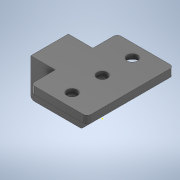
# Autodesk Inventor part: pulleysupport2
Saved by Autodesk Inventor 2020.2 (Build 242310000, 310)
## iProperties
Created: 2020-08-06
Part Number: pulleysupport2
Material: Generic
Document SubType Name: Modeling
Designer: JK
Density: 1 g/cm^3
Appearance: Smooth - Black
Author: JK
Autodesk Inventor part; units mm, degrees
ref_plane "YZ Plane" through (0, 0, 0) normal (1, 0, 0) x (0, 1, 0)
ref_plane "XZ Plane" through (0, 0, 0) normal (0, 1, 0) x (-1, 0, 0)
ref_plane "XY Plane" through (0, 0, 0) normal (0, 0, 1) x (1, 0, 0)
sketch "Sketch1" plane through (0, 0, 0) normal (0, 1, 0) x (-1, 0, 0)
  line L0 (-15, 23) -> (15, 23)
  line L1 (15, 23) -> (15, -23)
  line L2 (15, -23) -> (-15, -23)
  line L3 (-15, -23) -> (-15, 23)
  line L4 (-15, 23) -> (15, -23) construction
  line L5 (15, 23) -> (-15, -23) construction
  circle A0 centre (0, 16) radius 1.75
  circle A1 centre (0, -16) radius 1.75
  point P0 (0, 0)
  dimension "d0" = 3.5
  dimension "d1" = 30
  dimension "d2" = 46
  dimension "d3" = 16
  dimension "d4" = 16
  constraints: 12 end point, 2 centre point, 2 midpoint, 2 parallel, 1 equal radius, 1 horizontal, 1 perpendicular
  measures "d0" diameter of A0
  measures "d1" distance of L0.start L0.end
  measures "d2" distance of L0.end L1.end
  measures "d3" distance of A0.centre point (0, 0)
  measures "d4" distance of A1.centre point (0, 0)
extrude "Extrusion1" add sketch "Sketch1" along normal blind 4
sketch "Sketch2" plane through (0, 4, 0) normal (0, 1, 0) x (1, 0, 0)
  line L0 (15, -23) -> (15, 23) projected
  line L1 (15, -10) -> (-28, -10)
  line L2 (-28, -10) -> (-28, 10)
  line L3 (-28, 10) -> (15, 10)
  line L4 (15, 10) -> (15, -10)
  line L5 (-15, -23) -> (15, -23) projected
  point P0 (0, 0)
  point P1 (15, 10)
  dimension "d9" = 20
  dimension "d11" = 10
  dimension "d28" = 43
  constraints: 8 end point, 2 parallel, 1 horizontal, 1 perpendicular, 1 point on line
  measures "d9" distance between parallel lines of L1 L3
  measures "d11" distance from line of L1 point (0, 0)
  measures "d28" distance between parallel lines of L0 L2
extrude "Extrusion2" add sketch "Sketch2" against normal blind 20
sketch "Sketch3" plane through (0, -16, 0) normal (0, -1, 0) x (1, 0, 0)
  point P0 (0, 0)
sketch "Sketch4" plane through (0, -16, 0) normal (0, -1, 0) x (1, 0, 0)
  line L0 (35.8206, -4.75) -> (-35.8206, -4.75)
  line L1 (-35.8206, -4.75) -> (-35.8206, 4.75)
  line L2 (-35.8206, 4.75) -> (35.8206, 4.75)
  line L3 (35.8206, 4.75) -> (35.8206, -4.75)
  line L4 (35.8206, -4.75) -> (-35.8206, 4.75) construction
  line L5 (-35.8206, -4.75) -> (35.8206, 4.75) construction
  point P0 (0, 0)
  dimension "d12" = 9.5
  constraints: 12 end point, 2 midpoint, 2 parallel, 1 horizontal, 1 perpendicular
  measures "d12" distance between parallel lines of L2 L0
extrude "Extrusion3" cut sketch "Sketch4" against normal up to surface (16 mm away)
sketch "Sketch5" plane through (-15, 4, -10) normal (0, 0, -1) x (-1, 0, 0)
  circle A0 centre (8, -15) radius 1.5
  line L0 (13, 0) -> (13, -20) projected
  line L1 (13, -20) -> (-30, -20) projected
  point P0 (-15, -4)
  dimension "d15" = 3
  dimension "d16" = 5
  dimension "d17" = 5
  constraints: 1 centre point
  measures "d15" diameter of A0
  measures "d16" distance from line of L0 A0.centre
  measures "d17" distance from line of A0.centre L1
extrude "Extrusion4" cut sketch "Sketch5" against normal through all
sketch "Sketch6" plane through (0, 0, 0) normal (0, -1, 0) x (1, 0, 0)
  circle A0 centre (0, -16) radius 1.75 projected
  circle A1 centre (0, -16) radius 4.75
  circle A2 centre (0, 16) radius 1.75 projected
  circle A3 centre (0, 16) radius 4.75
  point P0 (0, 0)
  dimension "d20" = 9.5
  dimension "d21" = 9.5
  constraints: 2 centre point, 2 coincident
  measures "d20" diameter of A1
  measures "d21" diameter of A3
extrude "Extrusion5" cut sketch "Sketch6" against normal blind 2
fillet "Fillet1" radius 2 6 edges at (-15, 2, -23) (15, 2, -23) (-15, 2, 23) (15, 2, 23) (-28, -16, -7.375) (-28, -16, 7.375)
chamfer "Chamfer1" distance 16 angle 45 2 edges at (15, -16, -7.375) (15, -16, 7.375)
fillet "Fillet2" radius 2 2 edges at (-1, -16, 7.375) (-1, -16, -7.375)
fillet "Fillet3" radius 2 2 edges at (-6.5, 0, -4.75) (-6.5, 0, 4.75)
fillet "Fillet4" radius 2 2 edges at (0, 0, 10) (0, 0, -10)
sketch "Sketch7" plane through (-28, 4, 10) normal (0, 0, 1) x (1, 0, 0)
  point P0 (28, -4)
  point P1 (5, -15)
sketch "Sketch8" plane through (-28, 0, 2.75) normal (0, -1, 0) x (1, 0, 0)
  circle A0 centre (28, -2.75) radius 4.75
  dimension "d32" = 9.5
  constraints: 1 centre point, 1 coincident
  measures "d32" diameter of A0
extrude "Extrusion6" cut sketch "Sketch8" along normal blind 20.5 and the other way blind 2
sketch "Sketch9" plane through (0, 2, 0) normal (0, -1, 0) x (1, 0, 0)
  circle A0 centre (0, 0) radius 2.75
  circle A1 centre (0, -16) radius 1.75 projected
  circle A2 centre (0, -16) radius 2.75
  circle A3 centre (0, 16) radius 1.75 projected
  circle A4 centre (0, 16) radius 2.75
  dimension "d37" = 5.5
  constraints: 3 centre point, 3 coincident, 2 equal radius
  measures "d37" diameter of A0
extrude "Extrusion7" cut sketch "Sketch9" against normal blind 10
sketch "Sketch10" plane through (-1.8284, -16, 4.75) normal (0, 0, -1) x (-1, 0, 0)
  circle A0 centre (21.1716, 5) radius 1.5 projected
  circle A1 centre (21.1716, 5) radius 2.15
  point P0 (-1.8284, 16)
  dimension "d40" = 4.3
  constraints: 1 centre point, 1 coincident
  measures "d40" diameter of A1
extrude "Extrusion8" add sketch "Sketch10" along normal blind 10
sketch "Sketch11" plane through (0, -16, 0) normal (0, -1, 0) x (1, 0, 0)
  line L0 (-31.2906, 4.35) -> (-15.1457, 4.35)
  line L1 (-15.1457, 4.35) -> (-15.1457, -4.35)
  line L2 (-15.1457, -4.35) -> (-31.2906, -4.35)
  line L3 (-31.2906, -4.35) -> (-31.2906, 4.35)
  line L4 (-26, 4.75) -> (-1.8284, 4.75) projected
  line L5 (-1.8284, -4.75) -> (-26, -4.75) projected
  point P0 (0, 0)
  dimension "d45" = 0.4
  dimension "d46" = 0.4
  constraints: 8 end point, 2 parallel, 1 horizontal, 1 perpendicular
  measures "d45" distance between parallel lines of L4 L0
  measures "d46" distance between parallel lines of L5 L2
extrude "Extrusion9" cut sketch "Sketch11" against normal blind 9.25
body "Solid1"
